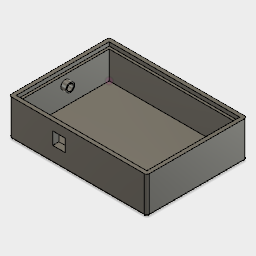
LED_bottom (Autodesk Fusion 360 design; units mm, degrees)
Autodesk Fusion 360 part; units mm, degrees
sketch "Sketch1" plane through (0, 0, 0) normal (0, 1, 0) x (1, 0, 0)
sketch "Sketch2" plane through (0, 0, 0) normal (0, 1, 0) x (1, 0, 0)
  line L0 (0, 0) -> (110, 0)
  line L1 (110, 0) -> (110, -80)
  line L2 (110, -80) -> (0, -80)
  line L3 (0, -80) -> (0, 0)
extrude "Extrude1" add sketch "Sketch2" along normal blind 30
shell "Shell2" thickness 5 removed faces 1 at (36.6667, 30, 26.6667)
fillet "Fillet6" radius 2 7 edges at (55, 0, 80) (110, 15, 80) (110, 0, 40) (0, 0, 40) (55, 0, 0) (0, 15, 80) (110, 15, 0)
fillet "Fillet7" radius 2 2 edges at (0.5858, 0.5858, 0.5858) (0, 16, 0)
sketch "Sketch3" plane through (0, 0, 0) normal (-1, 0, 0) x (0, 0, 1)
  line L0 (2, 30) -> (2, 2)
  line L1 (2, 2) -> (78, 2)
  line L2 (78, 2) -> (78, 30)
  line L3 (78, 30) -> (2, 30)
  circle A0 centre (40, 20) radius 2.55
sketch "Sketch6" plane through (0, 0, 80) normal (0, 0, 1) x (1, 0, 0)
  line L0 (108, 2) -> (108, 30)
  line L1 (108, 30) -> (2, 30)
  line L2 (2, 30) -> (2, 2)
  line L3 (2, 2) -> (108, 2)
  line L4 (45, 13) -> (35, 13)
  line L5 (35, 13) -> (35, 23)
  line L6 (35, 23) -> (45, 23)
  line L7 (45, 23) -> (45, 13)
  line L8 (45, 13) -> (35, 23) construction
  line L9 (35, 13) -> (45, 23) construction
  point P0 (40, 18)
extrude "Extrude3" cut sketch "Sketch6" against normal blind 5 contours L4 L5 L6 L7
sketch "Sketch10" plane through (0, 30, 0) normal (0, 1, 0) x (-1, 0, 0)
  arc A0 (-2, 0) -> (0, 2) centre (-2, 2) ccw
  line L0 (0, 2) -> (0, 78)
  arc A1 (0, 78) -> (-2, 80) centre (-2, 78) ccw
  line L1 (-2, 80) -> (-108, 80)
  arc A2 (-108, 80) -> (-110, 78) centre (-108, 78) ccw
  line L2 (-110, 78) -> (-110, 2)
  arc A3 (-110, 2) -> (-108, 0) centre (-108, 2) ccw
  line L3 (-108, 0) -> (-2, 0)
  line L4 (-5, 75) -> (-5, 5)
  line L5 (-5, 5) -> (-105, 5)
  line L6 (-105, 5) -> (-105, 75)
  line L7 (-105, 75) -> (-5, 75)
  line L8 (-3, 3) -> (-107, 3)
  line L9 (-107, 3) -> (-107, 77)
  line L10 (-107, 77) -> (-3, 77)
  line L11 (-3, 77) -> (-3, 3)
extrude "Extrude4" cut sketch "Sketch10" along normal mid plane 6 contours L8 L9 L10 L11
extrude "Extrude5" cut sketch "Sketch3" along normal mid plane 20 contours A0
fillet "Fillet9" radius 2 1 edges at (0, 20.9221, 37.6226)
sketch "Sketch12" plane through (5, 0, 0) normal (1, 0, 0) x (0, 0, -1)
  circle A0 centre (-40, 20) radius 2.55
  line L0 (-5, 27) -> (-75, 27)
  line L1 (-75, 27) -> (-75, 5)
  line L2 (-75, 5) -> (-5, 5)
  line L3 (-5, 5) -> (-5, 27)
  circle A1 centre (-40, 20) radius 3.5
extrude "Extrude6" add sketch "Sketch12" along normal blind 4 contours A1
